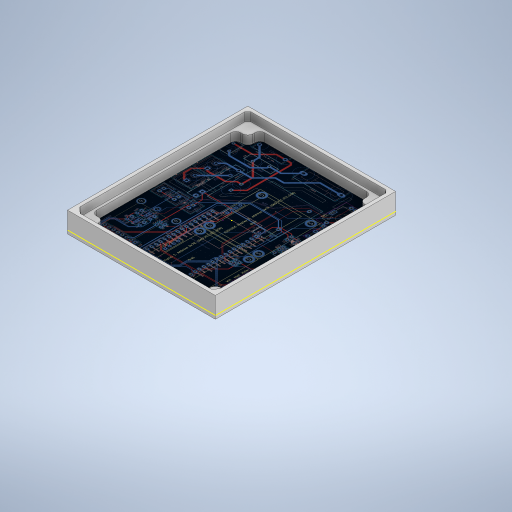
# Autodesk Inventor part: box
Saved by Autodesk Inventor 2024 (Build 280153000, 153)
## iProperties
Created: 2026-03-02
Part Number: box
Material: Generic
Document SubType Name: Modeling
Designer: Emil
Density: 1 g/cm^3
Appearance: Default
Author: Emil
Autodesk Inventor part; units mm, degrees
ref_plane "YZ Plane" through (0, 0, 0) normal (1, 0, 0) x (0, 1, 0)
ref_plane "XZ Plane" through (0, 0, 0) normal (0, 1, 0) x (-1, 0, 0)
ref_plane "XY Plane" through (0, 0, 0) normal (0, 0, 1) x (1, 0, 0)
sketch "Sketch1" plane through (0, 0, 0) normal (0, 1, 0) x (-1, 0, 0)
  line L0 (41, 50.45) -> (40.9472, -50.4928) construction
  line L1 (40.9472, -50.4928) -> (-41, -50.45) construction
  line L2 (-41, -50.45) -> (-40.9472, 50.4928) construction
  line L3 (-40.9472, 50.4928) -> (41, 50.45) construction
  line L4 (-41, 50.45) -> (41, -50.45) construction
  line L5 (41, 50.45) -> (-41, -50.45) construction
  line L6 (-43, 52.45) -> (43, 52.45)
  line L7 (43, 52.45) -> (43, -52.45)
  line L8 (43, -52.45) -> (-43, -52.45)
  line L9 (-43, -52.45) -> (-43, 52.45)
  line L10 (-43, 52.45) -> (43, -52.45) construction
  line L11 (43, 52.45) -> (-43, -52.45) construction
  line L12 (41, 50.45) -> (41, 50.0105)
  line L13 (41.001, 46.9167) -> (41.001, -48.4427)
  line L14 (41, -50.45) -> (40.9473, -50.45)
  line L15 (39.0158, -50.4509) -> (-38.9625, -50.4509)
  line L16 (-38.3742, 50.45) -> (37.4278, 50.45)
  line L17 (-40.999, -48.5131) -> (-40.9487, 47.6278)
  line L18 (37.4278, 50.45) -> (37.7432, 50.4517)
  line L19 (41.001, 46.9167) -> (41.0014, 47.2908)
  line L20 (41.0014, 47.2908) -> (37.7432, 50.4517)
  line L21 (41.001, -48.4427) -> (41.001, -48.6823)
  line L22 (41.001, -48.6823) -> (39.229, -50.4509)
  line L23 (39.229, -50.4509) -> (39.0158, -50.4509)
  line L24 (-38.9625, -50.4509) -> (-39.191, -50.4509)
  line L25 (-39.191, -50.4509) -> (-40.9991, -48.7299)
  line L26 (-40.999, -48.5131) -> (-40.9991, -48.7299)
  line L27 (-40.9487, 47.6278) -> (-40.9486, 47.9339)
  line L28 (-38.3742, 50.45) -> (-38.6199, 50.45)
  line L29 (-38.6199, 50.45) -> (-40.9486, 47.9339)
  point P0 (0, 0)
  dimension "d48" = 82
  dimension "d49" = 100.9
  dimension "d50" = 86
  dimension "d51" = 104.9
  constraints: 52 end point, 7 point on line, 4 midpoint, 4 parallel, 4 perpendicular, 3 horizontal, 2 coincident, 2 collinear, 1 vertical, 3 other
  measures "d48" distance of L4.end L5.end
  measures "d49" distance of L5.start L4.end
  measures "d50" distance of L7.end L8.end
  measures "d51" distance of L6.end L7.end
extrude "Extrusion3" add sketch "Sketch1" along normal blind 10
sketch "Sketch3" plane through (0, 0, 0) normal (0, -1, 0) x (1, 0, 0)
  line L0 (43, -52.45) -> (-43, -52.45) projected
  line L1 (-43, 52.45) -> (43, 52.45)
  line L2 (43, 52.45) -> (43, -52.45)
  line L3 (43, -52.45) -> (-43, -52.45)
  line L4 (-43, -52.45) -> (-43, 52.45)
  line L5 (-43, 52.45) -> (43, -52.45) construction
  line L6 (43, 52.45) -> (-43, -52.45) construction
  point P0 (0, 0)
  constraints: 12 end point, 2 midpoint, 2 parallel, 1 horizontal, 1 perpendicular
extrude "Extrusion4" add sketch "Sketch3" along normal blind 2
sketch "Sketch4" plane through (0, 0, 0) normal (0, 1, 0) x (1, 0, 0)
  line L0 (-40.966, -50.4517) -> (-40.966, 50.4509) construction
  line L1 (-40.966, 50.4509) -> (40.9486, 50.4509) construction
  line L2 (40.9486, 50.4509) -> (40.9486, -50.4517) construction
  line L3 (40.9486, -50.4517) -> (-40.966, -50.4517) construction
  line L4 (-41.001, -46.9167) -> (-41.001, 48.6823) projected
  line L5 (-37.7432, -50.4517) -> (-41.0014, -47.2908) projected
  line L6 (38.6199, -50.45) -> (-37.4278, -50.45) projected
  line L7 (43, 52.45) -> (-43, 52.45) projected
  line L8 (-43, 52.45) -> (-43, -52.45) projected
  line L9 (-43, -52.45) -> (43, -52.45) projected
  line L10 (43, -52.45) -> (43, 52.45) projected
  line L11 (-41.0014, -47.2908) -> (-41.001, -46.9167) projected
  line L12 (-41.001, -46.9167) -> (-41.001, 48.6823) projected
  line L13 (-41.001, 48.6823) -> (-39.229, 50.4509) projected
  line L14 (-39.229, 50.4509) -> (38.9625, 50.4509) projected
  line L15 (38.9625, 50.4509) -> (39.191, 50.4509) projected
  line L16 (39.191, 50.4509) -> (40.9991, 48.7299) projected
  line L17 (40.9991, 48.7299) -> (40.9486, -47.9339) projected
  line L18 (40.9486, -47.9339) -> (38.6199, -50.45) projected
  line L19 (38.6199, -50.45) -> (-37.4278, -50.45) projected
  line L20 (-37.4278, -50.45) -> (-37.7432, -50.4517) projected
  line L21 (-37.7432, -50.4517) -> (-41.0014, -47.2908) projected
  line L22 (-39.229, 50.4509) -> (38.9625, 50.4509) projected
  line L23 (-41.001, 48.6823) -> (-39.229, 50.4509) projected
  point P0 (0, 0)
  constraints: 2 other
sketch "Sketch5" plane through (0, 0, 0) normal (0, 1, 0) x (1, 0, 0)
  line L0 (-37.7432, -50.4517) -> (-41.0014, -47.2908) projected
  line L1 (-37.4278, -50.45) -> (-37.7432, -50.4517) projected
  line L2 (38.6199, -50.45) -> (-37.4278, -50.45) projected
  line L3 (40.9486, -47.9339) -> (38.6199, -50.45) projected
  line L4 (40.9991, 48.7299) -> (40.9486, -47.9339) projected
  line L5 (39.191, 50.4509) -> (40.9991, 48.7299) projected
  line L6 (38.9625, 50.4509) -> (39.191, 50.4509) projected
  line L7 (-39.229, 50.4509) -> (38.9625, 50.4509) projected
  line L8 (-41.001, 48.6823) -> (-39.229, 50.4509) projected
  line L9 (-41.001, -46.9167) -> (-41.001, 48.6823) projected
  line L10 (-41.0014, -47.2908) -> (-41.001, -46.9167) projected
  line L11 (-37.7432, -50.4517) -> (-41.0014, -47.2908) projected
  line L12 (38.6199, -50.45) -> (-37.4278, -50.45) projected
  line L13 (-37.4278, -50.45) -> (-37.7432, -50.4517) projected
  line L14 (-41.001, -46.9167) -> (-41.001, 48.6823) projected
  line L15 (-41.0014, -47.2908) -> (-41.001, -46.9167) projected
  line L16 (-41.001, 48.6823) -> (-39.229, 50.4509) projected
  line L17 (-39.229, 50.4509) -> (38.9625, 50.4509) projected
  line L18 (39.191, 50.4509) -> (40.9991, 48.7299) projected
  line L19 (40.9991, 48.7299) -> (40.9486, -47.9339) projected
  line L20 (40.9486, -47.9339) -> (38.6199, -50.45) projected
  line L21 (-41.0014, -47.2908) -> (-40.9669, 48.7164)
  line L22 (-39.229, 50.4509) -> (39.191, 50.4509)
  line L23 (40.9485, 48.778) -> (40.9486, -47.9339)
  line L24 (38.6199, -50.45) -> (-37.7432, -50.4517)
  line L25 (-37.7432, -50.4517) -> (-41.0014, -47.2908)
  line L26 (39.5283, -48.9788) -> (-39.5283, -48.9788)
  line L27 (-39.5283, -48.9788) -> (-39.5283, 48.9788)
  line L28 (-39.5283, 48.9788) -> (39.5283, 48.9788)
  line L29 (39.5283, 48.9788) -> (39.5283, -48.9788)
  line L30 (39.5283, -48.9788) -> (-39.5283, 48.9788) construction
  line L31 (-39.5283, -48.9788) -> (39.5283, 48.9788) construction
  line L32 (-39.5283, -48.9788) -> (-32.5283, -48.9788)
  line L33 (-32.5283, -48.9788) -> (-32.5283, -41.9788)
  line L34 (-32.5283, -41.9788) -> (-39.5283, -41.9788)
  line L35 (-39.5283, -41.9788) -> (-39.5283, -48.9788)
  line L36 (-39.5283, 48.9788) -> (-32.5283, 48.9788)
  line L37 (-32.5283, 48.9788) -> (-32.5283, 41.9788)
  line L38 (-32.5283, 41.9788) -> (-39.5283, 41.9788)
  line L39 (-39.5283, 41.9788) -> (-39.5283, 48.9788)
  line L40 (39.5283, 48.9788) -> (32.5283, 48.9788)
  line L41 (32.5283, 48.9788) -> (32.5283, 41.9788)
  line L42 (32.5283, 41.9788) -> (39.5283, 41.9788)
  line L43 (39.5283, 41.9788) -> (39.5283, 48.9788)
  line L44 (39.5283, -48.9788) -> (32.5283, -48.9788)
  line L45 (32.5283, -48.9788) -> (32.5283, -41.9788)
  line L46 (32.5283, -41.9788) -> (39.5283, -41.9788)
  line L47 (39.5283, -41.9788) -> (39.5283, -48.9788)
  point P0 (0, 0)
  point P1 (-41.001, -46.1517)
  point P2 (-39.5283, -48.7199)
  point P3 (-39.2615, -48.9788)
  dimension "d152" = 7
  dimension "d153" = 7
  dimension "d154" = 7
  dimension "d155" = 7
  dimension "d156" = 7
  dimension "d157" = 7
  dimension "d158" = 7
  dimension "d159" = 7
  constraints: 54 end point, 10 parallel, 6 perpendicular, 5 horizontal, 2 midpoint, 2 point on line
  measures "d152" distance of L34.end L33.end
  measures "d153" distance of L33.end L32.end
  measures "d154" distance of L37.end L38.end
  measures "d155" distance of L36.end L37.end
  measures "d156" distance of L42.end L41.end
  measures "d157" distance of L41.end L40.end
  measures "d158" distance of L45.end L46.end
  measures "d159" distance of L44.end L45.end
extrude "Extrusion5" add sketch "Sketch5" along normal blind 5 contours L0 L26 L29 L28 L27 L10 L21 L8 L7 L6 L5 L23 L3 L2 L1 | L0 L27 L34 L33 L26 | L45 L46 L29 L26 | L27 L28 L37 L38 | L42 L41 L28 L29
fillet "Fillet1" radius 3 12 edges at (-39.5283, 2.5, 41.9788) (-32.5283, 2.5, 41.9788) (-32.5283, 2.5, 48.9788) (-32.5283, 2.5, -48.9788) (-32.5283, 2.5, -41.9788) (-39.5283, 2.5, -41.9788) (32.5283, 2.5, -48.9788) (32.5283, 2.5, -41.9788) (39.5283, 2.5, -41.9788) (39.5283, 2.5, 41.9788) (32.5283, 2.5, 41.9788) (32.5283, 2.5, 48.9788)
body "Solid2"
